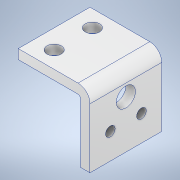
# Autodesk Inventor part: Soporte de Final de Carrera - Eje X
Saved by Autodesk Inventor 2020 (Build 240168000, 168)
## iProperties
Created: 2020-05-23
Part Number: Soporte de Final de Carrera - Eje X
Material: Aluminum 1100-H14
Document SubType Name: Modeling
Designer: Dante
Density: 2.7 g/cm^3
Appearance: Aluminum - Flat
Author: Dante
Autodesk Inventor part; units mm, degrees
ref_plane "YZ Plane" through (0, 0, 0) normal (1, 0, 0) x (0, 1, 0)
ref_plane "XZ Plane" through (0, 0, 0) normal (0, 1, 0) x (-1, 0, 0)
ref_plane "XY Plane" through (0, 0, 0) normal (0, 0, 1) x (1, 0, 0)
sketch "Sketch1" plane through (0, 0, 0) normal (0, 0, 1) x (1, 0, 0)
  line L0 (3, 0) -> (3, -15)
  line L1 (3, -15) -> (1, -15)
  line L2 (1, -15) -> (1, -2)
  line L3 (1, -2) -> (-12, -2)
  line L4 (-12, -2) -> (-12, 0)
  line L5 (-12, 0) -> (3, 0)
  line L6 (-12, 0) -> (3, 0)
  dimension "d38" = 2
  dimension "d39" = 13
  dimension "d40" = 13
  dimension "d41" = 2
  constraints: 14 end point, 4 perpendicular, 1 collinear, 1 parallel, 1 vertical
  measures "d38" distance of L0.end L1.end
  measures "d39" distance of L1.end L2.end
  measures "d40" distance of L2.end L3.end
  measures "d41" distance of L3.end L4.end
extrude "Extrusion3" add sketch "Sketch1" along normal blind 15
sketch "Sketch2" plane through (-12, -2, 0) normal (0, -1, 0) x (1, 0, 0)
  circle A0 centre (4, 3.5) radius 1.5
  line L0 (0, 15) -> (13, 15) projected
  line L1 (0, 0) -> (0, 15) projected
  line L2 (0, 0) -> (13, 0) projected
  circle A1 centre (4, 11.5) radius 1.5
  dimension "d45" = 3
  dimension "d47" = 4
  dimension "d48" = 3.5
  dimension "d49" = 3
  dimension "d50" = 4
  dimension "d51" = 3.5
  constraints: 2 centre point
  measures "d45" diameter of A0
  measures "d47" distance from line of L1 A0.centre
  measures "d48" distance from line of L2 A0.centre
  measures "d49" diameter of A1
  measures "d50" distance from line of L1 A1.centre
  measures "d51" distance from line of L0 A1.centre
extrude "Extrusion4" cut sketch "Sketch2" against normal blind 10
sketch "Sketch3" plane through (1, -15, 0) normal (-1, 0, 0) x (0, 0, 1)
  circle A0 centre (10.75, 5.375) radius 1
  circle A1 centre (4.25, 5.375) radius 1
  line L0 (0, 0) -> (15, 0) projected
  line L1 (15, 13) -> (15, 0) projected
  line L2 (0, 13) -> (0, 0) projected
  circle A2 centre (7.5, 10) radius 2
  dimension "d54" = 2
  dimension "d55" = 2
  dimension "d56" = 5.375
  dimension "d57" = 5.375
  dimension "d58" = 4.25
  dimension "d59" = 4.25
  dimension "d62" = 4
  dimension "d65" = 10
  constraints: 3 centre point
  measures "d54" diameter of A0
  measures "d55" diameter of A1
  measures "d56" distance from line of A0.centre L0
  measures "d57" distance from line of A1.centre L0
  measures "d58" distance from line of L1 A0.centre
  measures "d59" distance from line of L2 A1.centre
  measures "d62" diameter of A2
  measures "d65" distance from line of L0 A2.centre
extrude "Extrusion5" cut sketch "Sketch3" against normal blind 10 contours A0 | A1
extrude "Extrusion6" cut sketch "Sketch3" against normal blind 10 contours A2
fillet "Fillet1" radius 2.5 1 edges at (3, 0, 7.5)
fillet "Fillet2" radius 0.5 1 edges at (1, -2, 7.5)
equation "\"d51\" = d48"
equation "\"d58\" = d59"
body "Solid3"
